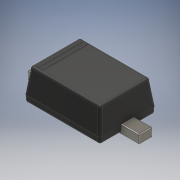
# Autodesk Inventor part: Semiconductor_DO219AB
Saved by Autodesk Inventor 2018 (Build 220112000, 112)
## iProperties
Created: 2018-09-29
Part Number: Semiconductor_DO219AB
Material: ABS Plastic
Document SubType Name: Modeling
Designer: Bradley
Density: 1.06 g/cm^3
Appearance: Smooth - Black
Author: Bradley
Autodesk Inventor part; units mm, degrees
ref_plane "YZ Plane" through (0, 0, 0) normal (1, 0, 0) x (0, 1, 0)
ref_plane "XZ Plane" through (0, 0, 0) normal (0, 1, 0) x (-1, 0, 0)
ref_plane "XY Plane" through (0, 0, 0) normal (0, 0, 1) x (1, 0, 0)
sketch "Sketch1" plane through (0, 0, 0) normal (0, 0, 1) x (1, 0, 0)
  line L0 (-0.85, -0.625) -> (0.85, -0.625)
  line L1 (0.85, -0.625) -> (0.85, 0.625)
  line L2 (0.85, 0.625) -> (-0.85, 0.625)
  line L3 (-0.85, 0.625) -> (-0.85, -0.625)
  line L4 (-0.85, -0.625) -> (0.85, 0.625) construction
  line L5 (0.85, -0.625) -> (-0.85, 0.625) construction
  point P0 (0, 0)
  dimension "d0" = 1.7
  dimension "d1" = 1.25
  constraints: 12 end point, 2 midpoint, 2 parallel, 1 horizontal, 1 perpendicular
  measures "d0" distance of L2.end L1.end
  measures "d1" distance of L1.end L0.end
extrude "Extrusion1" add sketch "Sketch1" along normal blind 0.55 draft -7 and the other way blind 0.15 draft -3
sketch "Sketch2" plane through (0, 0, 0) normal (0, 0, 1) x (1, 0, 0)
  line L0 (-0.7825, -0.5575) -> (-0.7825, 0.5575) projected
  line L1 (-0.85, 0.625) -> (-0.7825, 0.5575) projected
  line L2 (-0.85, 0.625) -> (-0.85, -0.625) projected
  line L3 (-0.85, -0.625) -> (-0.7825, -0.5575) projected
  line L4 (-0.7825, 0.5575) -> (0.7825, 0.5575) projected
  line L5 (0.85, 0.625) -> (0.7825, 0.5575) projected
  line L6 (0.85, 0.625) -> (-0.85, 0.625) projected
  line L7 (-0.85, 0.625) -> (-0.7825, 0.5575) projected
  line L8 (0.7825, 0.5575) -> (0.7825, -0.5575) projected
  line L9 (0.85, -0.625) -> (0.7825, -0.5575) projected
  line L10 (0.85, -0.625) -> (0.85, 0.625) projected
  line L11 (0.85, 0.625) -> (0.7825, 0.5575) projected
  line L12 (0.7825, -0.5575) -> (-0.7825, -0.5575) projected
  line L13 (-0.85, -0.625) -> (-0.7825, -0.5575) projected
  line L14 (-0.85, -0.625) -> (0.85, -0.625) projected
  line L15 (0.85, -0.625) -> (0.7825, -0.5575) projected
  line L16 (-1.25, 0.15) -> (-0.74, 0.15)
  line L17 (-0.74, 0.15) -> (-0.74, -0.15)
  line L18 (-0.74, -0.15) -> (-1.25, -0.15)
  line L19 (-1.25, -0.15) -> (-1.25, 0.15)
  line L20 (1.25, 0.15) -> (0.74, 0.15)
  line L21 (0.74, 0.15) -> (0.74, -0.15)
  line L22 (0.74, -0.15) -> (1.25, -0.15)
  line L23 (1.25, -0.15) -> (1.25, 0.15)
  line L24 (-1.25, 0) -> (1.25, 0) construction
  point P0 (0, 0)
  point P1 (0, 0)
  dimension "d6" = 0.3
  dimension "d7" = 2.5
  dimension "d8" = 0.51
  constraints: 18 end point, 4 parallel, 3 collinear, 3 midpoint, 2 horizontal, 2 perpendicular, 1 coincident
  measures "d6" distance of L18.end L16.start
  measures "d7" distance between parallel lines of L23 L19
  measures "d8" distance of L16.start L16.end
extrude "Extrusion2" add sketch "Sketch2" against normal blind 0.175 and the other way blind 0.025 contours L18 L2 L16 L0 | L0 L16 L17 L18 | L18 L19 L16 L2 | L22 L21 L20 L8 | L8 L20 L10 L22 | L10 L20 L23 L22
sketch "Sketch3" plane through (0, 0, 0.55) normal (0, 0, 1) x (1, 0, 0)
  line L0 (-0.7, 0.5) -> (-0.65, 0.5)
  line L1 (-0.65, 0.5) -> (-0.65, -0.5)
  line L2 (-0.65, -0.5) -> (-0.7, -0.5)
  line L3 (-0.7, -0.5) -> (-0.7, 0.5)
  line L4 (-0.6, 0.5) -> (-0.55, 0.5)
  line L5 (-0.55, 0.5) -> (-0.55, -0.5)
  line L6 (-0.55, -0.5) -> (-0.6, -0.5)
  line L7 (-0.6, -0.5) -> (-0.6, 0.5)
  point P0 (0, 0)
  point P1 (-0.55, 0)
  dimension "d11" = 0.05
  dimension "d12" = 0.05
  dimension "d13" = 1
  dimension "d14" = 0.55
  constraints: 16 end point, 4 parallel, 2 horizontal, 2 perpendicular, 2 point on line, 1 collinear, 1 horizontal alignment, 1 midpoint
  measures "d11" distance of L4.start L4.end
  measures "d12" distance between parallel lines of L7 L1
  measures "d13" distance of L4.end L5.end
  measures "d14" distance from line of L5 point (0, 0)
extrude "Extrusion3" add sketch "Sketch3" along normal blind 0.01
fillet "Fillet1" radius 0.05 18 edges at (-0.8162, -0.5912, 0.275) (-0.8461, -0.6211, -0.075) (-0.7825, 0, 0.55) (0, -0.5575, 0.55) (0, 0.5575, 0.55) (-0.8162, 0.5912, 0.275) (-0.8461, 0.6211, -0.075) (-0.8421, 0.3836, -0.15) (0, 0.6171, -0.15) (-0.8421, -0.3836, -0.15) (0, -0.6171, -0.15) (0.8421, -0.3836, -0.15) (0.8461, -0.6211, -0.075) (0.8162, -0.5912, 0.275) (0.7825, 0, 0.55) (0.8421, 0.3836, -0.15) (0.8461, 0.6211, -0.075) (0.8162, 0.5912, 0.275)
fillet "Fillet2" radius 0.02 18 edges at (1.0485, 0.15, 0.025) (1.25, 0, 0.025) (1.0485, -0.15, 0.025) (1.25, -0.15, -0.075) (1.25, 0, -0.175) (0.995, 0.15, -0.175) (1.25, 0.15, -0.075) (0.74, 0, -0.175) (0.995, -0.15, -0.175) (-1.25, 0, -0.175) (-0.995, -0.15, -0.175) (-1.25, -0.15, -0.075) (-1.0485, -0.15, 0.025) (-1.25, 0, 0.025) (-0.995, 0.15, -0.175) (-1.25, 0.15, -0.075) (-0.74, 0, -0.175) (-1.0485, 0.15, 0.025)
equation "\"d12\" = d11"
body "Solid1"
